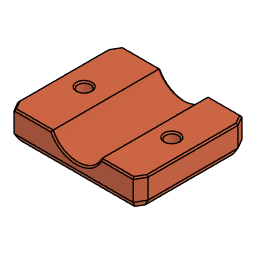
[a]_z_bearing_clamp_x4 (Autodesk Fusion 360 design; units mm, degrees)
Autodesk Fusion 360 part; units mm, degrees
note: some values were not read from the file. Set by a fixed rule: which sketch regions a step uses.
sketch "Sketch1" plane through (0, 0, 0) normal (0, 0, 1) x (1, 0, 0)
  line L0 (17.925, -15) -> (-17.925, -15)
  line L1 (-17.925, -15) -> (-17.925, 15)
  line L2 (-17.925, 15) -> (17.925, 15)
  line L3 (17.925, 15) -> (17.925, -15)
  line L4 (17.925, -15) -> (-17.925, 15) construction
  line L5 (-17.925, -15) -> (17.925, 15) construction
  line L6 (0, 0) -> (0, 15)
  line L7 (-16.425, 15) -> (-17.925, 12.4019)
  line L8 (16.425, 15) -> (17.925, 12.4019)
  line L9 (0, 0) -> (-17.925, 0)
  line L10 (-16.425, -15) -> (-17.925, -12.4019)
  line L11 (16.425, -15) -> (17.925, -12.4019)
  circle A0 centre (-12.1, 0) radius 1.75
  circle A1 centre (12.1, 0) radius 1.75
  circle A2 centre (-12.1, 0) radius 3.25
  circle A3 centre (12.1, 0) radius 3.25
  line L12 (-13.85, 2.7386) -> (-13.85, -2.7386)
  line L13 (-10.35, 2.7386) -> (-10.35, -2.7386)
  line L14 (-13.85, 1.75) -> (-10.35, 1.75)
  line L15 (-10.35, -1.75) -> (-13.85, -1.75)
  line L16 (13.85, 1.75) -> (10.35, 1.75)
  line L17 (10.35, 2.7386) -> (10.35, -2.7386)
  line L18 (10.35, -1.75) -> (13.85, -1.75)
  line L19 (13.85, 2.7386) -> (13.85, -2.7386)
  line L20 (0, 0) -> (0, -15)
  dimension "d1" = 35.85
  dimension "d2" = 30
  dimension "d4" = 60
  dimension "d5" = 1.5
  dimension "d6" = 3.5
  dimension "d7" = 5.825
  dimension "d8" = 6.5
  constraint horizontal L0
  constraint perpendicular L0 L1
  constraint parallel L0 L2
  constraint parallel L1 L3
  constraint coincident L4 L6.start
  constraint coincident L5 L6.start
  constraint coincident L6.start L9.start
  constraint midpoint L2 L6.end
  constraint coincident L2 L7.start
  constraint coincident L1 L7.end
  constraint symmetric L6 L7.start L8.start
  constraint symmetric L6 L7.end L8.end
  constraint midpoint L1 L9.end
  constraint symmetric L7.start L9 L10.start
  constraint symmetric L7.end L9 L10.end
  constraint symmetric L6 L10.start L11.start
  constraint symmetric L6 L10.end L11.end
  constraint coincident L9 A0.centre
  constraint symmetric L6 A0 A1
  constraint concentric A0 A2
  constraint symmetric L6 A2 A3
  constraint coincident A2 L12.start
  constraint coincident A2 L12.end
  constraint vertical L13
  constraint vertical L12
  constraint tangent A0 L12
  constraint tangent A0 L13
  constraint coincident L12 L14.start
  constraint coincident L13 L15.start
  constraint coincident L12 L15.end
  constraint coincident A2 L13.end
  constraint horizontal L15
  constraint horizontal L14
  constraint tangent A0 L14
  constraint tangent A0 L15
  constraint coincident A2 L13.start
  constraint coincident L13 L14.end
  constraint symmetric L6 L12.start L19.start
  constraint symmetric L6 L12.end L19.end
  constraint symmetric L6 L13.start L17.start
  constraint symmetric L6 L13.end L17.end
  constraint symmetric L6 L14.start L16.start
  constraint symmetric L6 L14.end L16.end
  constraint symmetric L6 L15.start L18.start
  constraint symmetric L6 L15.end L18.end
  constraint coincident L0 L20.end
  constraint vertical L20
  measures "d1" distance of L1.end L2.end
  measures "d2" distance of L0.end L1.end
  measures "d4" angle of L2 L7
  measures "d5" distance of L1.end L7.start
  measures "d6" diameter of A0
  measures "d7" distance of L1 A0.centre
  measures "d8" diameter of A2
extrude "Extrude1" add sketch "Sketch1" along normal blind 7.6 contours L0 L2 L3 L6 L8 L11 L20 | L0 L1 L9 L10 A2 L20 | L1 L2 L6 L7 L9 A2 | L9 A2 L13 | L9 A2 L13 | A0 L13 L15 | A0 L13 L14 | A2 L12 L13 L14 | A2 L12 L13 L15 | L9 A2 L12 | L9 A2 L12 | A0 L12 L14 | A0 L12 L15 | A1 L18 L19 | A1 L16 L19 | A3 L19 | A3 L16 L17 L19 | A1 L16 L17 | A1 L17 L18 | A3 L17 L18 L19 | A3 L17
extrude "Extrude5" cut sketch "Sketch1" against normal blind 3.6 from surface at 7.6 contours A0 L13 L15 | A0 L13 L14 | A0 L12 L14 | A0 L12 L15 | A1 L18 L19 | A1 L16 L19 | A1 L16 L17 | A1 L17 L18
extrude "Extrude6" cut sketch "Sketch1" against normal blind 3.3 from surface at 7.6 contours A2 L12 L13 L14 | A2 L12 L13 L15 | A3 L16 L17 L19 | A3 L17 L18 L19
extrude "Extrude7" cut sketch "Sketch1" against normal blind 3 from surface at 7.6 contours L9 A2 L13 | L9 A2 L13 | L9 A2 L12 | L9 A2 L12 | A3 L19 | A3 L17
chamfer "Chamfer1" distance 1 angle 60 8 edges at (-17.925, 0, 7.6) (-17.175, -13.701, 7.6) (-17.175, 13.701, 7.6) (0, 15, 7.6) (17.175, 13.701, 7.6) (17.925, 0, 7.6) (17.175, -13.701, 7.6) (0, -15, 7.6) measured on face at (-3.3967, -10.8765, 7.6) measured on face at (-3.3967, -10.8765, 7.6) measured on face at (-3.3967, -10.8765, 7.6) measured on face at (-3.3967, -10.8765, 7.6) measured on face at (-3.3967, -10.8765, 7.6) measured on face at (-3.3967, -10.8765, 7.6) measured on face at (-3.3967, -10.8765, 7.6) measured on face at (-3.3967, -10.8765, 7.6)
hole "Hole1" at (0.725, 15, -3.25) direction (0, -1, 0) diameter 15 depth 30 tip angle 180
chamfer "Chamfer4" distance 0.4 angle 45 14 edges at (-13.7316, -0.6328, 0) (-11.2296, 15, 0) (0.725, 15, 4.25) (11.9546, 15, 0) (17.175, 13.701, 0) (17.925, 0, 0) (17.175, -13.701, 0) (11.9546, -15, 0) (0.725, -15, 4.25) (-11.2296, -15, 0) (-17.175, -13.701, 0) (10.4684, -0.6328, 0) (-17.925, 0, 0) (-17.175, 13.701, 0)
chamfer "Chamfer5" distance 0.4 angle 45 2 edges at (-15.1301, 1.1753, 7.6) (9.0699, 1.1753, 7.6)
move_body "Move1" bodies 1 to x (1, 0, 0) y (0, -1, 0) z (0, 0, -1) at (0, 0, 0)
move_body "Move2" bodies 1 to x (1, 0, 0) y (0, 1, 0) z (0, 0, 1) at (0, 0, 7.6)
equation "d9 = 10.6 mm - 3 mm"
